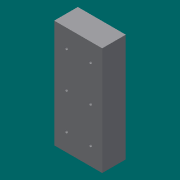
# Autodesk Inventor part: 知能ロボコンスペーサ1.1
Saved by Autodesk Inventor 2013 (Build 170138000, 138)
## iProperties
Created: 2014-11-22
Part Number: 知能ロボコンスペーサ1.1
Material: 一般
Document SubType Name: Modeling
Designer: horumo136
Density: 1 g/cm^3
Author: horumo136
Autodesk Inventor part; units mm, degrees
ref_plane "YZ Plane" through (0, 0, 0) normal (1, 0, 0) x (0, 1, 0)
ref_plane "XZ Plane" through (0, 0, 0) normal (0, 1, 0) x (-1, 0, 0)
ref_plane "XY Plane" through (0, 0, 0) normal (0, 0, 1) x (1, 0, 0)
sketch "スケッチ1" plane through (0, 0, 0) normal (0, 1, 0) x (-1, 0, 0)
  line L0 (0, 0) -> (40, 0)
  line L1 (40, 0) -> (40, 90)
  line L2 (40, 90) -> (0, 90)
  line L3 (0, 90) -> (0, 0)
  line L4 (0, 90) -> (10, 90)
  line L5 (10, 90) -> (10, 76.25)
  line L6 (10, 75) -> (0, 75)
  line L7 (0, 75) -> (0, 90)
  line L8 (40, 90) -> (30, 90)
  line L9 (30, 90) -> (30, 76.25)
  line L10 (30, 75) -> (40, 75)
  line L11 (40, 75) -> (40, 90)
  line L12 (0, 0) -> (10, 0)
  line L13 (10, 0) -> (10, 13.75)
  line L14 (10, 15) -> (0, 15)
  line L15 (0, 15) -> (0, 0)
  line L16 (40, 0) -> (30, 0)
  line L17 (30, 0) -> (30, 13.75)
  line L18 (30, 15) -> (40, 15)
  line L19 (40, 15) -> (40, 0)
  circle A0 centre (10, 75) radius 1.25
  circle A1 centre (30, 75) radius 1.25
  circle A2 centre (10, 45) radius 1.25
  circle A3 centre (30, 45) radius 1.25
  circle A4 centre (10, 15) radius 1.25
  circle A5 centre (30, 15) radius 1.25
  dimension "d10" = 2.5
  dimension "d11" = 2.5
  dimension "d14" = 2.5
  dimension "d15" = 2.5
  dimension "d0" = 40
  dimension "d1" = 90
  dimension "d2" = 10
  dimension "d3" = 15
  dimension "d4" = 10
  dimension "d5" = 15
  dimension "d6" = 10
  dimension "d7" = 15
  dimension "d8" = 10
  dimension "d9" = 15
  dimension "d12" = 2.5
  dimension "d13" = 2.5
  constraints: 40 end point, 10 parallel, 6 coincident, 5 horizontal, 5 perpendicular, 4 vertical alignment, 2 centre point, 8 other
  measures "d0" distance of L2.end L1.end
  measures "d1" distance of L1.end L0.end
  measures "d2" distance of L6.start L6.end
  measures "d3" distance of L4.end L6.start
  measures "d4" distance of L10.end L10.start
  measures "d5" distance of L10.start L8.end
  measures "d6" distance of L14.end L14.start
  measures "d7" distance of L14.start L12.end
  measures "d8" distance of L18.start L18.end
  measures "d9" distance of L16.end L18.start
  measures "d12" diameter of A2
  measures "d13" diameter of A3
extrude "押し出し1" add sketch "スケッチ1" along normal blind 19.7 contours L3 L14 A4 L13 L0 | L13 A4 L14 L3 L6 A0 L5 L2 L9 A1 L10 L1 L18 A5 L17 L0 | L17 A5 L18 L1 L0 | L3 L2 L5 A0 L6 | L10 A1 L9 L2 L1
